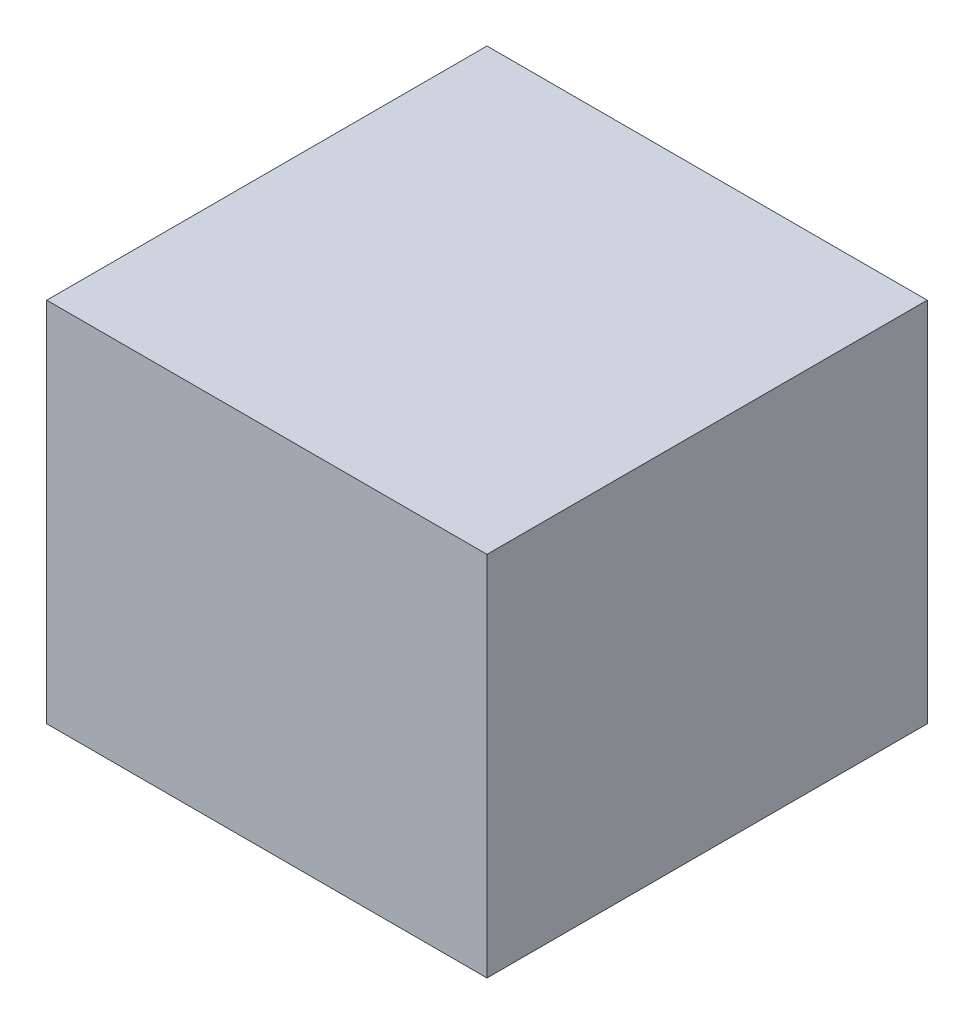
# Autodesk Inventor part: Эскиз рама
Saved by Autodesk Inventor 2025 (Build 290162010, 162A)
## iProperties
Created: 2024-09-30
Part Number: Эскиз рама
Material: Generic
Document SubType Name: Modeling
Designer: pokla
Density: 1 g/cm^3
Appearance: Default
Author: pokla
Autodesk Inventor part; units mm, degrees
ref_plane "YZ Plane" through (0, 0, 0) normal (1, 0, 0) x (0, 1, 0)
ref_plane "XZ Plane" through (0, 0, 0) normal (0, 1, 0) x (-1, 0, 0)
ref_plane "XY Plane" through (0, 0, 0) normal (0, 0, 1) x (1, 0, 0)
sketch "Sketch1" plane through (0, 0, 0) normal (0, 1, 0) x (-1, 0, 0)
  line L0 (-900, 900) -> (900, 900)
  line L1 (900, 900) -> (900, -900)
  line L2 (900, -900) -> (-900, -900)
  line L3 (-900, -900) -> (-900, 900)
  line L4 (-900, -900) -> (900, 900) construction
  point P0 (0, 0)
  point P1 (0, 0)
  dimension "d0" = 1800
  dimension "d1" = 1800
  constraints: 10 end point, 2 parallel, 1 coincident, 1 horizontal, 1 midpoint, 1 perpendicular
  measures "d0" distance of L0.start L0.end
  measures "d1" distance of L2.end L0.start
extrude "Extrusion1" add sketch "Sketch1" along normal blind 1500
body "Solid1"
